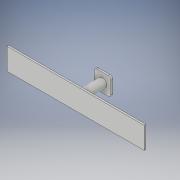
# Autodesk Inventor part: Hot Shoe Mount
Saved by Autodesk Inventor 2018 (Build 220112000, 112)
## iProperties
Created: 2018-08-14
Part Number: Hot Shoe Mount
Material: Generic
Document SubType Name: Modeling
Designer: F8PLTW
Density: 1 g/cm^3
Appearance: Default
Author: F8PLTW
Autodesk Inventor part; units mm, degrees
ref_plane "YZ Plane" through (0, 0, 0) normal (1, 0, 0) x (0, 1, 0)
ref_plane "XZ Plane" through (0, 0, 0) normal (0, 1, 0) x (-1, 0, 0)
ref_plane "XY Plane" through (0, 0, 0) normal (0, 0, 1) x (1, 0, 0)
sketch "Sketch1" plane through (0, 0, 0) normal (0, 0, 1) x (1, 0, 0)
  line L0 (-2.2587, 5.9544) -> (9.9913, 5.9544)
  line L1 (13.1663, 2.7794) -> (13.1663, -10.8706)
  line L2 (9.9913, -14.0456) -> (-2.2587, -14.0456)
  line L3 (-5.4337, -10.8706) -> (-5.4337, 2.7794)
  arc A0 (13.1663, 2.7794) -> (9.9913, 5.9544) centre (9.9913, 2.7794) ccw
  arc A1 (9.9913, -14.0456) -> (13.1663, -10.8706) centre (9.9913, -10.8706) ccw
  arc A2 (-5.4337, -10.8706) -> (-2.2587, -14.0456) centre (-2.2587, -10.8706) ccw
  arc A3 (-2.2587, 5.9544) -> (-5.4337, 2.7794) centre (-2.2587, 2.7794) ccw
  point P0 (0, 0)
  point P1 (13.1663, -14.0456)
  point P2 (13.1663, 5.9544)
  point P3 (-5.4337, -14.0456)
  dimension "d0" = 18.6
  dimension "d1" = 20
  dimension "d2" = 3.175
  constraints: 8 end point, 8 point on circle, 8 tangent, 6 point on line, 4 centre point, 3 equal radius, 2 parallel, 1 horizontal, 1 perpendicular
  measures "d0" distance of point (13.166, -14.046) point (-5.434, -14.046)
  measures "d1" distance of point (13.166, 5.954) point (13.166, -14.046)
  measures "d2" radius of A0
extrude "Extrusion1" add sketch "Sketch1" along normal blind 2
sketch "Sketch2" plane through (0, 0, 2) normal (0, 0, 1) x (1, 0, 0)
  arc A0 (-2.2587, 5.9544) -> (-5.4337, 2.7794) centre (-2.2587, 2.7794) ccw projected
  arc A1 (9.9913, -14.0456) -> (13.1663, -10.8706) centre (9.9913, -10.8706) ccw projected
  line L0 (-2.2587, 2.7794) -> (9.9913, -10.8706) construction
  arc A2 (13.1663, 2.7794) -> (9.9913, 5.9544) centre (9.9913, 2.7794) ccw projected
  arc A3 (-5.4337, -10.8706) -> (-2.2587, -14.0456) centre (-2.2587, -10.8706) ccw projected
  line L1 (9.9913, 2.7794) -> (-2.2587, -10.8706) construction
  circle A4 centre (3.8663, -4.0456) radius 4.7625
  point P0 (0, 0)
  dimension "d5" = 9.525
  constraints: 4 end point, 1 centre point, 1 midpoint
  measures "d5" diameter of A4
extrude "Extrusion2" add sketch "Sketch2" along normal blind 28
sketch "Sketch3" plane through (3.8663, -4.0456, 30) normal (0, 0, 1) x (1, 0, 0)
  line L0 (-76.2, -12.065) -> (76.2, -12.065)
  line L1 (76.2, -12.065) -> (76.2, 12.065)
  line L2 (76.2, 12.065) -> (-76.2, 12.065)
  line L3 (-76.2, 12.065) -> (-76.2, -12.065)
  line L4 (-76.2, -12.065) -> (76.2, 12.065) construction
  line L5 (76.2, -12.065) -> (-76.2, 12.065) construction
  point P0 (-3.8663, 4.0456)
  point P1 (0, 0)
  point P2 (0, 0)
  dimension "d8" = 24.13
  dimension "d9" = 152.4
  constraints: 12 end point, 3 midpoint, 2 parallel, 1 horizontal, 1 perpendicular
  measures "d8" distance of L1.end L0.end
  measures "d9" distance of L1.end L2.end
extrude "Extrusion3" add sketch "Sketch3" along normal blind 2
body "Solid1"
